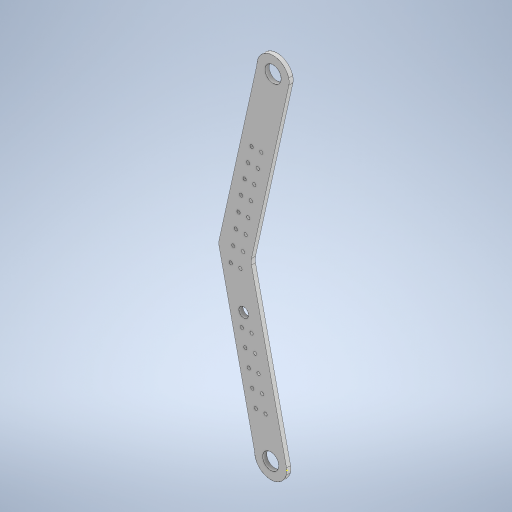
# Autodesk Inventor part: angle v3 inside
Saved by Autodesk Inventor 2023 (Build 270158000, 158)
## iProperties
Created: 2023-02-07
Part Number: angle v3 inside
Material: Generic
Document SubType Name: Modeling
Designer: Wyatt
Density: 1 g/cm^3
Appearance: Default
Author: Wyatt
Autodesk Inventor part; units mm, degrees
ref_plane "YZ Plane" through (0, 0, 0) normal (1, 0, 0) x (0, 1, 0)
ref_plane "XZ Plane" through (0, 0, 0) normal (0, 1, 0) x (-1, 0, 0)
ref_plane "XY Plane" through (0, 0, 0) normal (0, 0, 1) x (1, 0, 0)
sketch "Sketch1" plane through (0, 0, 0) normal (0, 0, 1) x (1, 0, 0)
  line L0 (0, 0) -> (-24.739, 111.5906)
  line L1 (0, 0) -> (114.3, 0) construction
  line L2 (-24.739, 111.5906) -> (0, 223.1813)
  line L3 (0, 223.1813) -> (-25.4, 223.1813)
  line L4 (-24.739, 111.5906) -> (-50.139, 111.5906)
  line L5 (0, 0) -> (-25.4, 0)
  line L6 (-25.4, 0) -> (-50.139, 111.5906)
  line L7 (-25.4, 223.1813) -> (-50.139, 111.5906)
  arc A0 (0, 223.1813) -> (-25.4, 223.1813) centre (-12.7, 223.1813) ccw
  arc A1 (-25.4, 0) -> (0, 0) centre (-12.7, 0) ccw
  circle A2 centre (-12.7, 0) radius 6.35
  circle A3 centre (-12.7, 223.1813) radius 6.35
  line L8 (0, 0) -> (-28.396, 128.086)
  line L9 (-28.396, 128.086) -> (1.8406, 264.4745)
  line L10 (-28.396, 128.086) -> (111.304, 128.086) construction
  line L11 (1.8406, 264.4745) -> (-23.5594, 264.4745)
  line L12 (-28.396, 128.086) -> (-53.796, 128.086)
  line L13 (-53.796, 128.086) -> (-23.5594, 264.4745)
  line L14 (0, 0) -> (-25.4, 0)
  line L15 (-53.796, 128.086) -> (-25.4, 0)
  arc A4 (-25.4, 0) -> (0, 0) centre (-12.7, 0) ccw
  circle A5 centre (-12.7, 0) radius 6.35
  arc A6 (1.8406, 264.4745) -> (-23.5594, 264.4745) centre (-10.8594, 264.4745) ccw
  circle A7 centre (-10.8594, 264.4745) radius 6.35
  dimension "d0" = 114.3
  dimension "d1" = 102.5
  dimension "d2" = 114.3
  dimension "d3" = 155
  dimension "d4" = 25.4
  dimension "d5" = 25.4
  dimension "d6" = 25.4
  dimension "d7" = 12.7
  dimension "d8" = 12.7
  dimension "d9" = 12.7
  dimension "d10" = 12.7
  dimension "d24" = 139.7
  dimension "d25" = 77.5
  dimension "d26" = 25.4
  dimension "d27" = 25.4
  dimension "d28" = 12.7
  dimension "d29" = 12.7
  constraints: 32 end point, 8 centre point, 8 point on circle, 7 horizontal, 4 coincident, 2 concentric, 2 equal length, 1 collinear, 1 parallel, 1 point on line
  measures "d0" distance of L0.start L0.end
  measures "d1" angle of L1 L0
  measures "d2" distance of L0.end L2.end
  measures "d3" angle of L0 L2
  measures "d4" distance of L2.end L3.end
  measures "d5" distance of L0.end L4.end
  measures "d6" distance of L0.start L5.end
  measures "d7" radius of A0
  measures "d8" radius of A1
  measures "d9" diameter of A2
  measures "d10" diameter of A3
  measures "d24" distance of L8.end L9.end
  measures "d25" angle of L10 L9
  measures "d26" distance of L9.end L11.end
  measures "d27" distance of L8.end L12.end
  measures "d28" radius of A6
  measures "d29" diameter of A7
extrude "Extrusion3" add sketch "Sketch1" along normal blind 6.35 contours L5 A2 L6 L4 L0 | A1 L5 A2 | L4 L7 L12 L8 | L15 L12 L7 | L12 L7 L3 A3 L9 | L9 A3 L3 A0 | A0 L7 L12 L13 L11 A7 L9 | A3 L3 L9 | L3 A3 L9 | L11 A7 A6 picked at (-23.0997, 224.6964) picked at (-15.0808, 222.6929) picked at (-15.082, 223.6647)
sketch "Sketch3" plane through (0, 0, 6.35) normal (0, 0, 1) x (1, 0, 0)
  line L0 (1.8406, 264.4745) -> (-28.396, 128.086) projected
  line L1 (-53.796, 128.086) -> (-23.5594, 264.4745) projected
  line L2 (-28.396, 128.086) -> (-53.796, 128.086)
  line L3 (-28.396, 128.086) -> (-23.8337, 107.5068)
  line L4 (-28.396, 128.086) -> (0, 0) projected
  line L5 (-25.4, 0) -> (-53.796, 128.086) projected
  line L6 (-41.096, 128.086) -> (-36.3335, 103.1365)
  circle A0 centre (-10.8594, 264.4745) radius 6.35 projected
  line L7 (-41.096, 128.086) -> (-33.9522, 90.6617)
  line L8 (-41.096, 128.086) -> (-39.9054, 121.8486)
  line L9 (-41.096, 128.086) -> (-28.396, 128.086)
  line L10 (-41.096, 128.086) -> (-33.9522, 90.6617)
  line L11 (-33.9522, 90.6617) -> (-28.8722, 90.6617) construction
  circle A1 centre (-33.9522, 90.6617) radius 3.81
  line L12 (-38.6033, 115.0277) -> (-36.8935, 106.0705)
  line L13 (-35.4604, 115.6269) -> (-24.0304, 115.6269) construction
  circle A2 centre (-33.3166, 104.3997) radius 1.27
  dimension "d42" = 25.4
  dimension "d50" = 38.1
  dimension "d51" = 6.35
  dimension "d59" = 7.62
  dimension "d82" = 2.54
  constraints: 20 end point, 3 horizontal, 3 point on line, 2 centre point, 2 collinear, 1 coincident, 1 midpoint
  measures "d42" distance of L6.start L6.end
  measures "d50" distance of L6.start L7.end
  measures "d51" distance of L6.start L8.end
  measures "d59" diameter of A1
  measures "d82" diameter of A2
sketch "Sketch5" plane through (0, 0, 6.35) normal (0, 0, 1) x (1, 0, 0)
  circle A0 centre (-10.8594, 264.4745) radius 7.4295
  circle A1 centre (-12.7, 0) radius 7.4295
  point P0 (0, 0)
  dimension "d76" = 14.859
  dimension "d77" = 14.859
  constraints: 2 centre point, 2 coincident
  measures "d76" diameter of A0
  measures "d77" diameter of A1
extrude "Extrusion14" cut sketch "Sketch5" against normal blind 25.4
extrude "Extrusion15" cut sketch "Sketch3" against normal blind 25.4 contours A1 | A2
sketch "Sketch6" plane through (0, 0, 6.35) normal (0, 0, 1) x (1, 0, 0)
  circle A0 centre (-33.3166, 104.3997) radius 1.27 projected
  line L0 (0, 0) -> (-28.396, 128.086) projected
  line L1 (-33.3166, 104.3997) -> (-7.9166, 104.3997) construction
  line L2 (-33.3166, 104.3997) -> (-27.8191, 79.6018)
  line L3 (-33.3166, 104.3997) -> (-7.9166, 104.3997) construction
  line L4 (-27.8191, 79.6018) -> (-25.0703, 67.2029)
  line L5 (-25.0703, 67.2029) -> (-22.3215, 54.8039)
  line L6 (-22.3215, 54.8039) -> (-19.5727, 42.4049)
  line L7 (-19.5727, 42.4049) -> (-16.8239, 30.006)
  circle A1 centre (-27.8191, 79.6018) radius 1.27
  circle A2 centre (-25.0703, 67.2029) radius 1.27
  circle A3 centre (-22.3215, 54.8039) radius 1.27
  circle A4 centre (-19.5727, 42.4049) radius 1.27
  circle A5 centre (-16.8239, 30.006) radius 1.27
  dimension "d89" = 25.4
  dimension "d90" = 77.5
  dimension "d91" = 12.7
  dimension "d92" = 12.7
  dimension "d93" = 12.7
  dimension "d94" = 12.7
  dimension "d95" = 2.54
  dimension "d96" = 2.54
  dimension "d97" = 2.54
  dimension "d98" = 2.54
  dimension "d99" = 2.54
  constraints: 14 end point, 5 centre point, 5 coincident, 4 point on line, 2 horizontal, 1 equal length
  measures "d89" distance of L1.start L2.end
  measures "d90" angle of L2 L3
  measures "d91" distance of L2.end L4.end
  measures "d92" distance of L4.end L5.end
  measures "d93" distance of L5.end L6.end
  measures "d94" distance of L6.end L7.end
  measures "d95" diameter of A1
  measures "d96" diameter of A2
  measures "d97" diameter of A3
  measures "d98" diameter of A4
  measures "d99" diameter of A5
extrude "Extrusion16" cut sketch "Sketch6" against normal blind 25.4 contours A5 | A4 L7 L6 | L6 L7 A4 | A3 L6 L5 | L5 L6 A3 | A2 L5 L4 | L4 L5 A2 | A1 L4 L2 | L2 L4 A1
sketch "Sketch7" plane through (0, 0, 6.35) normal (0, 0, 1) x (1, 0, 0)
  circle A0 centre (-33.3166, 104.3997) radius 1.27 projected
  line L0 (-33.3166, 104.3997) -> (-36.559, 119.2908)
  circle A1 centre (-36.559, 119.2908) radius 1.27
  point P0 (0, 0)
  dimension "d102" = 15.24
  dimension "d103" = 2.54
  constraints: 2 end point, 1 centre point, 1 coincident
  measures "d102" distance of L0.start L0.end
  measures "d103" diameter of A1
extrude "Extrusion17" cut sketch "Sketch7" against normal blind 25.4 contours A1
sketch "Sketch8" plane through (0, 0, 6.35) normal (0, 0, 1) x (1, 0, 0)
  circle A0 centre (-36.559, 119.2908) radius 1.27 projected
  circle A1 centre (-22.3215, 54.8039) radius 1.27 projected
  circle A2 centre (-19.5727, 42.4049) radius 1.27 projected
  circle A3 centre (-25.0703, 67.2029) radius 1.27 projected
  circle A4 centre (-16.8239, 30.006) radius 1.27 projected
  circle A5 centre (-27.8191, 79.6018) radius 1.27 projected
  circle A6 centre (-33.9522, 90.6617) radius 3.81 projected
  circle A7 centre (-33.3166, 104.3997) radius 1.27 projected
  circle A8 centre (-10.8594, 264.4745) radius 7.4295 projected
  circle A9 centre (-12.7, 0) radius 7.4295 projected
  arc A10 (-25.4, 0) -> (0, 0) centre (-12.7, 0) ccw projected
  line L0 (-28.396, 128.086) -> (0, 0) projected
  line L1 (1.8406, 264.4745) -> (-28.396, 128.086) projected
  arc A11 (1.8406, 264.4745) -> (-23.5594, 264.4745) centre (-10.8594, 264.4745) ccw projected
  line L2 (-53.796, 128.086) -> (-23.5594, 264.4745) projected
  line L3 (-25.4, 0) -> (-53.796, 128.086) projected
extrude "Extrusion18" cut sketch "Sketch8" against normal blind 3.175
sketch "Sketch9" plane through (0, 0, 3.175) normal (0, 0, 1) x (1, 0, 0)
  circle A0 centre (-36.559, 119.2908) radius 1.27 projected
  line L0 (-36.559, 119.2908) -> (-28.396, 169.4307)
  line L1 (-36.559, 119.2908) -> (-44.179, 119.2908)
  circle A1 centre (-33.3166, 104.3997) radius 1.27 projected
  line L2 (-33.3166, 104.3997) -> (-40.9366, 104.3997)
  circle A2 centre (-27.8191, 79.6018) radius 1.27 projected
  line L3 (-27.8191, 79.6018) -> (-35.4391, 79.6018)
  circle A3 centre (-25.0703, 67.2029) radius 1.27 projected
  line L4 (-25.0703, 67.2029) -> (-32.6903, 67.2029)
  circle A4 centre (-22.3215, 54.8039) radius 1.27 projected
  line L5 (-22.3215, 54.8039) -> (-29.9415, 54.8039)
  circle A5 centre (-19.5727, 42.4049) radius 1.27 projected
  line L6 (-19.5727, 42.4049) -> (-27.1927, 42.4049)
  circle A6 centre (-16.8239, 30.006) radius 1.27 projected
  line L7 (-16.8239, 30.006) -> (-24.4439, 30.006)
  circle A7 centre (-27.1927, 42.4049) radius 1.27
  circle A8 centre (-24.4439, 30.006) radius 1.27
  circle A9 centre (-29.9415, 54.8039) radius 1.27
  circle A10 centre (-32.6903, 67.2029) radius 1.27
  circle A11 centre (-35.4391, 79.6018) radius 1.27
  circle A12 centre (-40.9366, 104.3997) radius 1.27
  circle A13 centre (-44.179, 119.2908) radius 1.27
  line L8 (-36.559, 119.2908) -> (-34.5183, 131.8258)
  line L9 (-34.5183, 131.8258) -> (-32.4775, 144.3607)
  line L10 (-32.4775, 144.3607) -> (-30.4367, 156.8957)
  line L11 (-28.396, 169.4307) -> (-25.6472, 181.8296)
  line L12 (-28.396, 169.4307) -> (-15.696, 169.4307) construction
  line L13 (-25.6472, 181.8296) -> (-22.8984, 194.2286)
  line L14 (-22.8984, 194.2286) -> (-20.1496, 206.6275)
  line L15 (-20.1496, 206.6275) -> (-27.7696, 206.6275)
  line L16 (-22.8984, 194.2286) -> (-30.5184, 194.2286)
  line L17 (-25.6472, 181.8296) -> (-33.2672, 181.8296)
  line L18 (-28.396, 169.4307) -> (-36.016, 169.4307)
  line L19 (-30.4367, 156.8957) -> (-38.0567, 156.8957)
  line L20 (-32.4775, 144.3607) -> (-40.0975, 144.3607)
  line L21 (-34.5183, 131.8258) -> (-42.1383, 131.8258)
  circle A14 centre (-27.7696, 206.6275) radius 1.27
  circle A15 centre (-20.1496, 206.6275) radius 1.27
  circle A16 centre (-30.5184, 194.2286) radius 1.27
  circle A17 centre (-22.8984, 194.2286) radius 1.27
  circle A18 centre (-33.2672, 181.8296) radius 1.27
  circle A19 centre (-25.6472, 181.8296) radius 1.27
  circle A20 centre (-36.016, 169.4307) radius 1.27
  circle A21 centre (-28.396, 169.4307) radius 1.27
  circle A22 centre (-42.1383, 131.8258) radius 1.27
  circle A23 centre (-40.0975, 144.3607) radius 1.27
  circle A24 centre (-38.0567, 156.8957) radius 1.27
  circle A25 centre (-34.5183, 131.8258) radius 1.27
  circle A26 centre (-32.4775, 144.3607) radius 1.27
  circle A27 centre (-30.4367, 156.8957) radius 1.27
  point P0 (0, 0)
  dimension "d108" = 50.8
  dimension "d109" = 7.62
  dimension "d110" = 7.62
  dimension "d111" = 7.62
  dimension "d112" = 7.62
  dimension "d113" = 7.62
  dimension "d114" = 7.62
  dimension "d115" = 7.62
  dimension "d116" = 2.54
  dimension "d117" = 2.54
  dimension "d118" = 2.54
  dimension "d119" = 2.54
  dimension "d120" = 2.54
  dimension "d121" = 2.54
  dimension "d122" = 2.54
  dimension "d123" = 12.7
  dimension "d124" = 12.7
  dimension "d125" = 12.7
  dimension "d126" = 12.7
  dimension "d127" = 77.5
  dimension "d128" = 12.7
  dimension "d129" = 12.7
  dimension "d130" = 7.62
  dimension "d131" = 7.62
  dimension "d132" = 7.62
  dimension "d133" = 7.62
  dimension "d134" = 7.62
  dimension "d135" = 7.62
  dimension "d136" = 7.62
  dimension "d137" = 2.54
  dimension "d138" = 2.54
  dimension "d139" = 2.54
  dimension "d140" = 2.54
  dimension "d141" = 2.54
  dimension "d142" = 2.54
  dimension "d143" = 2.54
  dimension "d144" = 2.54
  dimension "d145" = 2.54
  dimension "d146" = 2.54
  dimension "d147" = 2.54
  dimension "d148" = 2.54
  dimension "d149" = 2.54
  dimension "d150" = 2.54
  constraints: 44 end point, 21 centre point, 21 coincident, 15 horizontal, 4 point on line, 1 equal length, 1 midpoint
  measures "d108" distance of L0.start L0.end
  measures "d109" distance of L0.start L1.end
  measures "d110" distance of L2.start L2.end
  measures "d111" distance of L3.start L3.end
  measures "d112" distance of L4.start L4.end
  measures "d113" distance of L5.start L5.end
  measures "d114" distance of L6.start L6.end
  measures "d115" distance of L7.start L7.end
  measures "d116" diameter of A7
  measures "d117" diameter of A8
  measures "d118" diameter of A9
  measures "d119" diameter of A10
  measures "d120" diameter of A11
  measures "d121" diameter of A12
  measures "d122" diameter of A13
  measures "d123" distance of L0.start L8.end
  measures "d124" distance of L8.end L9.end
  measures "d125" distance of L9.end L10.end
  measures "d126" distance of L0.end L11.end
  measures "d127" angle of L12 L11
  measures "d128" distance of L11.end L13.end
  measures "d129" distance of L13.end L14.end
  measures "d130" distance of L14.end L15.end
  measures "d131" distance of L13.end L16.end
  measures "d132" distance of L11.end L17.end
  measures "d133" distance of L0.end L18.end
  measures "d134" distance of L10.end L19.end
  measures "d135" distance of L9.end L20.end
  measures "d136" distance of L8.end L21.end
  measures "d137" diameter of A14
  measures "d138" diameter of A15
  measures "d139" diameter of A16
  measures "d140" diameter of A17
  measures "d141" diameter of A18
  measures "d142" diameter of A19
  measures "d143" diameter of A20
  measures "d144" diameter of A21
  measures "d145" diameter of A22
  measures "d146" diameter of A23
  measures "d147" diameter of A24
  measures "d148" diameter of A25
  measures "d149" diameter of A26
  measures "d150" diameter of A27
extrude "Extrusion19" cut sketch "Sketch9" against normal blind 3.175 contours A13 | A22 | A23 | A24 | A20 | A18 | A16 | A14 | A15 L15 L14 | L14 L15 A15 | A17 L16 L13 | L13 L14 A17 | A19 L17 L11 | L11 L13 A19 | A21 L18 L0 | L0 L11 A21 | A27 L19 L0 | L0 A27 | A26 L20 L0 | L0 A26 | A25 L21 L0 | L0 A25 | L21 A25 L0 | L20 A26 L0 | L19 A27 L0 | L18 A21 L11 | L17 A19 L13 | L16 A17 L14 | A12 | A11 | A10 | A9 | A7 | A8
sketch "Sketch10" plane through (0, 0, 3.175) normal (0, 0, 1) x (1, 0, 0)
  circle A0 centre (-33.3166, 104.3997) radius 1.27 projected
  circle A1 centre (-33.3166, 104.3997) radius 1.27
  circle A2 centre (-40.9366, 104.3997) radius 1.27 projected
  circle A3 centre (-40.9366, 104.3997) radius 1.27
  point P0 (0, 0)
  constraints: 2 centre point, 2 coincident
extrude "Extrusion20" add sketch "Sketch10" against normal blind 3.175
sketch "Sketch11" plane through (0, 0, 3.175) normal (0, 0, 1) x (1, 0, 0)
  point P0 (0, 0)
sketch "Sketch12" plane through (0, 0, 3.175) normal (0, 0, 1) x (1, 0, 0)
  point P0 (0, 0)
fillet "Fillet1" radius 10.16 6 edges at (-25.4, 0, 1.5875) (0, 0, 1.5875) (-53.796, 128.086, 1.5875) (-28.396, 128.086, 1.5875) (1.8406, 264.4745, 1.5875) (-23.5594, 264.4745, 1.5875)
sketch "Sketch13" plane through (0, 0, 3.175) normal (0, 0, 1) x (1, 0, 0)
  point P0 (0, 0)
sketch "Sketch14" plane through (0, 0, 3.175) normal (0, 0, 1) x (1, 0, 0)
  circle A0 centre (-12.7, 0) radius 7.4295 projected
  circle A1 centre (-12.7, 0) radius 6.35
  circle A2 centre (-10.8594, 264.4745) radius 7.4295 projected
  circle A3 centre (-10.8594, 264.4745) radius 6.35
  circle A4 centre (-10.8594, 264.4745) radius 7.4295
  point P0 (0, 0)
  dimension "d156" = 12.7
  dimension "d157" = 12.7
  constraints: 3 centre point, 3 coincident
  measures "d156" diameter of A1
  measures "d157" diameter of A3
extrude "Extrusion21" add sketch "Sketch14" against normal blind 3.175
body "Solid3"
